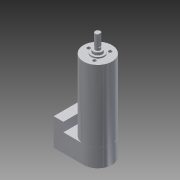
# Autodesk Inventor part: maxon_A-max22_110160
Saved by Autodesk Inventor 2015 (Build 190159000, 159)
## iProperties
Created: 2015-05-08
Part Number: maxon_A-max22_110160
Material: PVC、軟質
Document SubType Name: Modeling
Designer: kenta
Density: 2.90298 g/cm^3
Appearance: PVC - 白
Mass: 93 g
Surface Area: 73.6525 cm^2
Volume: 32.036 cm^3
Author: kenta
Autodesk Inventor part; units mm, degrees
ref_plane "YZ Plane" through (0, 0, 0) normal (1, 0, 0) x (0, 1, 0)
ref_plane "XZ Plane" through (0, 0, 0) normal (0, 1, 0) x (-1, 0, 0)
ref_plane "XY Plane" through (0, 0, 0) normal (0, 0, 1) x (1, 0, 0)
sketch "スケッチ1" plane through (0, 0, 0) normal (0, 0, 1) x (1, 0, 0)
  circle A0 centre (0, 0) radius 2
  dimension "d0" = 4
  constraints: 1 centre point, 1 coincident
  measures "d0" diameter of A0
extrude "押し出し1" add sketch "スケッチ1" along normal blind 11
sketch "スケッチ4" plane through (0, 0, 11) normal (0, 0, 1) x (1, 0, 0)
  line L0 (2, 0) -> (1.5, 0)
  line L1 (1.5, 0) -> (1.5, -1.5356)
  line L2 (1.5, -1.5356) -> (2, -1.5356)
  line L3 (2, -1.5356) -> (2, 0)
  point P0 (0, 0)
  dimension "d6" = 0.5
  constraints: 8 end point, 2 parallel, 1 horizontal, 1 perpendicular
  measures "d6" distance of L2.end L1.end
extrude "押し出し3" cut sketch "スケッチ4" against normal blind 9
sketch "スケッチ5" plane through (0, 0, 11) normal (0, 0, 1) x (1, 0, 0)
  circle A0 centre (0, 0) radius 2 projected
  line L0 (2, 0) -> (1.5, 0)
  line L1 (1.5, 0) -> (1.5, 4.3078)
  line L2 (1.5, 4.3078) -> (2, 4.3078)
  line L3 (2, 4.3078) -> (2, 0)
  dimension "d9" = 0.5
  constraints: 8 end point, 2 parallel, 1 horizontal, 1 horizontal alignment, 1 perpendicular, 1 other
  measures "d9" distance of L1.end L2.end
extrude "押し出し4" cut sketch "スケッチ5" against normal blind 9 contours L0 L1 A0 | A0 L1 L2 L3 picked at (1.5908, 0.7499)
sketch "スケッチ6" plane through (0, 0, 0) normal (0, 0, -1) x (-1, 0, 0)
  circle A0 centre (0, 0) radius 3.5
  dimension "d12" = 7
  constraints: 1 centre point, 1 coincident
  measures "d12" diameter of A0
extrude "押し出し5" add sketch "スケッチ6" along normal blind 2
sketch "スケッチ7" plane through (0, 0, -2) normal (0, 0, -1) x (-1, 0, 0)
  circle A0 centre (0, 0) radius 5
  dimension "d15" = 10
  constraints: 1 centre point, 1 coincident
  measures "d15" diameter of A0
extrude "押し出し6" add sketch "スケッチ7" along normal blind 1
sketch "スケッチ8" plane through (0, 0, -3) normal (0, 0, -1) x (-1, 0, 0)
  circle A0 centre (0, 0) radius 11
  dimension "d18" = 22
  constraints: 1 centre point, 1 coincident
  measures "d18" diameter of A0
extrude "押し出し7" add sketch "スケッチ8" along normal blind 55
sketch "スケッチ10" plane through (0, 0, -58) normal (0, 0, -1) x (-1, 0, 0)
  line L0 (11, 11) -> (-11, 11)
  line L1 (-11, 11) -> (-11, -11)
  line L2 (-11, -11) -> (11, -11)
  line L3 (11, -11) -> (11, 11)
  line L4 (11, 11) -> (-11, -11) construction
  line L5 (-11, 11) -> (11, -11) construction
  point P0 (0, 0)
  dimension "d21" = 22
  dimension "d22" = 22
  constraints: 12 end point, 2 midpoint, 2 parallel, 1 horizontal, 1 perpendicular
  measures "d21" distance of L2.end L1.end
  measures "d22" distance of L1.end L0.end
extrude "押し出し8" add sketch "スケッチ10" along normal blind 14
fillet "フィレット1" radius 10.9 1 edges at (11, -11, -65)
fillet "フィレット2" radius 10.9 1 edges at (11, 11, -65)
sketch "スケッチ13" plane through (-11, -11, -58) normal (-1, 0, 0) x (0, 0, 1)
  line L0 (0, 0) -> (-14, 0)
  line L1 (-14, 0) -> (-14, 22)
  line L2 (-14, 22) -> (0, 22)
  line L3 (0, 22) -> (0, 0)
  point P0 (58, 11)
  dimension "d27" = 14
  dimension "d28" = 22
  constraints: 8 end point, 2 parallel, 1 horizontal, 1 perpendicular
  measures "d27" distance of L1.end L2.end
  measures "d28" distance of L0.end L1.end
extrude "押し出し9" add sketch "スケッチ13" along normal blind 12
sketch "スケッチ14" plane through (0, 0, -58) normal (0, 0, 1) x (1, 0, 0)
  line L0 (-23, 11) -> (-15.5, 11)
  line L1 (-15.5, 11) -> (-15.5, -11)
  line L2 (-15.5, -11) -> (-23, -11)
  line L3 (-23, -11) -> (-23, 11)
  point P0 (0, 0)
  dimension "d31" = 7.5
  dimension "d32" = 22
  constraints: 8 end point, 2 parallel, 1 horizontal, 1 perpendicular
  measures "d31" distance of L1.end L2.end
  measures "d32" distance of L0.end L1.end
extrude "押し出し10" add sketch "スケッチ14" along normal blind 7
sketch "スケッチ16" plane through (0, 0, -3) normal (0, 0, 1) x (1, 0, 0)
  point P0 (0, 0)
  point P1 (-7, 0)
  dimension "d49" = 7
  dimension "d50" = 0
  measures "d49" distance of point (0, 0) point (-7, 0)
  measures "d50" vertical distance of point (0, 0) point (-7, 0)
hole "穴1" at (-7, 0, -3) direction (0, 0, -1) diameter 2.5 depth 4.5 tip angle 118
pattern_circular "円形状パターン2" count 3 over 360 about axis through (0, 0, 0) along (0, 0, 1) of "穴1"
